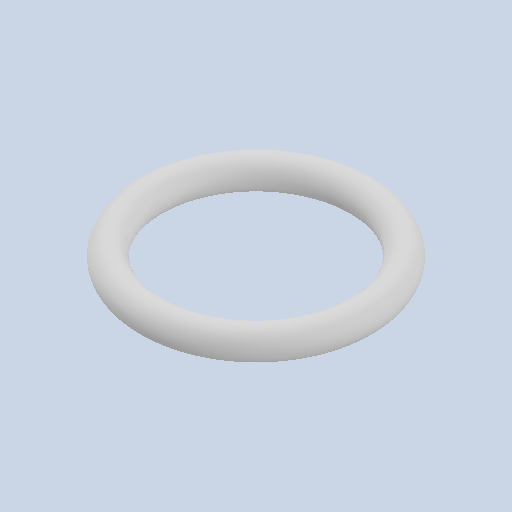
# Autodesk Inventor part: O'Ring 2-013
Saved by Autodesk Inventor 2025.3 (Build 293356030, 356C)
## iProperties
Created: 2024-04-18
Part Number: O'Ring 2-013
Material: Genérico
Document SubType Name: Modeling
Designer: santa
Density: 1 g/cm^3
Appearance: Valor por defecto
Author: santa
Autodesk Inventor part; units mm, degrees
ref_plane "YZ Plane" through (0, 0, 0) normal (1, 0, 0) x (0, 1, 0)
ref_plane "XZ Plane" through (0, 0, 0) normal (0, 1, 0) x (-1, 0, 0)
ref_plane "XY Plane" through (0, 0, 0) normal (0, 0, 1) x (1, 0, 0)
sketch "Boceto1" plane through (0, 0, 0) normal (0, 0, 1) x (1, 0, 0)
  circle A0 centre (6.3, 0) radius 0.89
  line L0 (0, 0) -> (0, 0)
  line L1 (0, 0) -> (6.3, 0) construction
  line L2 (0, -1.246) -> (0, 1.246) projected
  point P0 (5.41, 0)
  point P1 (7.19, 0)
  dimension "d0" = 1.78
  dimension "d3" = 10.82
  dimension "d4" = 14.38
  constraints: 4 end point, 2 horizontal alignment, 2 point on circle, 1 centre point, 1 horizontal, 1 midpoint, 1 perpendicular
  measures "d0" diameter of A0
  measures "d3" diameter of A0.start L0
  measures "d4" diameter of A0.end L0
revolve "Revolución1" add sketch "Boceto1" angle 360 about axis through (0, -10, 0) along (0, 1, 0)
